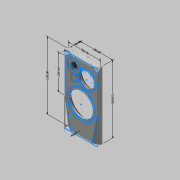
# Autodesk Inventor part: Front-panel
Saved by Autodesk Inventor 2022 (Build 260153070, 153G)
## iProperties
Created: 2021-11-16
Part Number: Front-panel
Material: Типовые
Document SubType Name: Modeling
Designer: kalugin_a
Density: 1 g/cm^3
Appearance: Белый дуб — натуральный — с умеренным глянцем
Author: kalugin_a
Autodesk Inventor part; units mm, degrees
ref_plane "YZ Plane" through (0, 0, 0) normal (1, 0, 0) x (0, 1, 0)
ref_plane "XZ Plane" through (0, 0, 0) normal (0, 1, 0) x (-1, 0, 0)
ref_plane "XY Plane" through (0, 0, 0) normal (0, 0, 1) x (1, 0, 0)
sketch "Эскиз1" plane through (0, 0, 0) normal (0, 0, 1) x (1, 0, 0)
  line L0 (125, 527.1036) -> (125, 6.4626) construction
  circle A0 centre (125, 228.3565) radius 93
  circle A1 centre (168.7833, 413.2707) radius 72.5
  circle A2 centre (67.9786, 456.6783) radius 51
  circle A3 centre (125, 228.3565) radius 110
  line L1 (52.0512, 396.4011) -> (83.9061, 396.4011)
  line L2 (88.9061, 391.4011) -> (88.9061, 359.1741)
  line L3 (83.9061, 354.1741) -> (52.0512, 354.1741)
  line L4 (47.0512, 359.1741) -> (47.0512, 391.4011)
  arc A4 (83.9061, 354.1741) -> (88.9061, 359.1741) centre (83.9061, 359.1741) ccw
  arc A5 (47.0512, 359.1741) -> (52.0512, 354.1741) centre (52.0512, 359.1741) ccw
  arc A6 (52.0512, 396.4011) -> (47.0512, 391.4011) centre (52.0512, 391.4011) ccw
  arc A7 (88.9061, 391.4011) -> (83.9061, 396.4011) centre (83.9061, 391.4011) ccw
  line L5 (0, 7.1036) -> (250, 7.1036)
  line L6 (250, 7.1036) -> (250, 527.1036)
  line L7 (250, 527.1036) -> (0, 527.1036)
  line L8 (0, 527.1036) -> (0, 7.1036)
  circle A8 centre (168.7833, 413.2707) radius 60
  circle A9 centre (67.9786, 456.6783) radius 25
  line L9 (0, 492.1036) -> (45, 527.1036)
  line L10 (205, 527.1036) -> (250, 492.1036)
  line L11 (0, 228.3565) -> (45, 7.1036)
  line L12 (250, 228.3565) -> (205, 7.1036)
  point P0 (106.0245, 471.357)
  point P1 (53.3, 494.7242)
  point P2 (29.9327, 441.9997)
  point P3 (82.6573, 418.6324)
  point P4 (196.0451, 456.6783)
  point P5 (144.8221, 458.584)
  point P6 (117.5603, 415.1763)
  point P7 (141.5215, 369.8631)
  point P8 (192.7445, 367.9575)
  point P9 (220.0063, 411.3651)
  point P10 (125, 328.8295)
  point P11 (53.9549, 299.4016)
  point P12 (24.527, 228.3565)
  point P13 (53.9549, 157.3114)
  point P14 (125, 127.8835)
  point P15 (196.0451, 157.3114)
  point P16 (225.473, 228.3565)
  point P17 (196.0451, 299.4016)
  point P18 (0, 0)
  dimension "d3" = 186
  dimension "d8" = 145
  dimension "d9" = 102
  dimension "d10" = 220
  dimension "d15" = 5
  dimension "d16" = 5
  dimension "d17" = 5
  dimension "d18" = 5
  dimension "d19" = 250
  dimension "d20" = 520
  dimension "d21" = 120
  dimension "d22" = 50
  dimension "d25" = 360
  dimension "d29" = 360
  dimension "d33" = 360
  dimension "d92" = 35
  dimension "d93" = 45
  dimension "d96" = 45
  dimension "d97" = 35
  dimension "d103" = 45
  dimension "d104" = 45
  dimension "d145" = 221.8939
  dimension "d146" = 406.8082
  dimension "d147" = 449.5747
  dimension "d148" = 81.2167
  dimension "d149" = 67.9786
  constraints: 26 end point, 10 centre point, 10 point on line, 8 point on circle, 8 tangent, 3 coincident, 2 parallel, 2 perpendicular, 1 horizontal, 1 midpoint, 1 vertical, 21 other
  measures "d3" diameter of A0
  measures "d8" diameter of A1
  measures "d9" diameter of A2
  measures "d10" diameter of A3
  measures "d15" radius of A4
  measures "d16" radius of A5
  measures "d17" radius of A6
  measures "d18" radius of A7
  measures "d19" distance of L6.end L7.end
  measures "d20" distance of L7.end L5.start
  measures "d21" diameter of A8
  measures "d22" diameter of A9
  measures "d92" distance of L7.end L9.start
  measures "d93" distance from line of L9.end L8
  measures "d96" distance of L10.start L6.end
  measures "d97" distance of L10.end L6.end
  measures "d103" distance of L12.end L5.end
  measures "d104" distance of L11.end L5.start
  measures "d145" distance of A0.centre L0.end
  measures "d146" vertical distance of A8.centre L0.end
  measures "d147" distance from line of L5 A2.centre
  measures "d148" distance from line of L6 A8.centre
  measures "d149" distance from line of L8 A2.centre
extrude "Выдавливание2" add sketch "Эскиз1" against normal blind 40 contours A1 A2 A8 | A2 A8 A1 | A1 A2 | A3 | L1 A7 L2 A4 L3 A5 L4 A6 | L8 L11 L5 | L11 L8 L9 L7 L10 L6 L12 L5 | L12 L6 L5 | L8 L7 L9 | L10 L7 L6
sketch "Эскиз3" plane through (0, 0, 0) normal (0, 0, 1) x (1, 0, 0)
  point P0 (0, 0)
  point P1 (53.2995, 494.7309)
  point P2 (29.4952, 442.4101)
  point P3 (82.4876, 418.8084)
  point P4 (105.644, 471.8009)
  point P5 (127.9097, 465.5665)
  point P6 (193.3079, 474.3405)
  point P7 (233.8339, 422.6329)
  point P8 (209.2871, 361.565)
  point P9 (144.1779, 352.2851)
  point P10 (103.6157, 404.0731)
  point P11 (83.8585, 391.5003)
  point P12 (51.9775, 391.5003)
  point P13 (51.8278, 359.3199)
  point P14 (83.7088, 359.3199)
  point P15 (124.8697, 328.9356)
  point P16 (53.9232, 299.4494)
  point P17 (24.437, 228.3533)
  point P18 (53.9232, 157.4068)
  point P19 (124.8697, 127.7709)
  point P20 (195.9659, 157.4068)
  point P21 (225.4521, 228.503)
  point P22 (195.9659, 299.5991)
hole "Отверстие1" at (53.2995, 494.7309, 0) at (29.4952, 442.4101, 0) at (82.4876, 418.8084, 0) at (105.644, 471.8009, 0) at (127.9097, 465.5665, 0) at (193.3079, 474.3405, 0) at (233.8339, 422.6329, 0) at (209.2871, 361.565, 0) at (144.1779, 352.2851, 0) at (103.6157, 404.0731, 0) at (83.8585, 391.5003, 0) at (51.9775, 391.5003, 0) at (51.8278, 359.3199, 0) at (83.7088, 359.3199, 0) at (124.8697, 328.9356, 0) at (53.9232, 299.4494, 0) at (24.437, 228.3533, 0) at (53.9232, 157.4068, 0) at (124.8697, 127.7709, 0) at (195.9659, 157.4068, 0) at (225.4521, 228.503, 0) at (195.9659, 299.5991, 0) direction (0, 0, -1) diameter 5 end through all counterbore diameter 6 counterbore depth 5
sketch "Эскиз4" plane through (0, 0, 0) normal (0, 0, 1) x (1, 0, 0)
  circle A0 centre (124.9966, 228.3645) radius 109.8136
  circle A1 centre (168.7833, 413.2703) radius 72.3983
  circle A2 centre (67.9786, 456.6783) radius 50.8827
  point P0 (0, 0)
  point P1 (118.17, 465.0372)
  point P2 (96.395, 414.4698)
  constraints: 3 centre point
extrude "Выдавливание3" cut sketch "Эскиз4" against normal blind 4
sketch "Эскиз6" plane through (0, 0, -4) normal (0, 0, 1) x (1, 0, 0)
  point P0 (0, 0)
  point P1 (78.9885, 479.1235)
  dimension "d3" = 186
  dimension "d8" = 145
  dimension "d9" = 102
  dimension "d10" = 220
  dimension "d19" = 250
  dimension "d20" = 520
  dimension "d21" = 120
  dimension "d22" = 50
  dimension "d25" = 360
  dimension "d29" = 360
  dimension "d33" = 360
  dimension "d92" = 35
  dimension "d93" = 45
  dimension "d96" = 45
  dimension "d97" = 35
  dimension "d103" = 45
  dimension "d104" = 45
  dimension "d145" = 221.8939
  dimension "d146" = 406.8082
  dimension "d147" = 449.5747
  dimension "d148" = 81.2167
  dimension "d149" = 67.9786
hole "Отверстие3" at (78.9885, 479.1235, -4) direction (0, 0, -1) diameter 15 end through all
sketch "Эскиз7" plane through (0, 0, -4) normal (0, 0, 1) x (1, 0, 0)
  point P0 (0, 0)
  point P1 (58.1005, 433.7127)
hole "Отверстие4" at (58.1005, 433.7127, -4) direction (0, 0, -1) diameter 15 end through all
sketch "Эскиз8" plane through (0, 0, 0) normal (0, 0, 1) x (1, 0, 0)
  line L0 (52.0512, 396.4011) -> (83.9061, 396.4011)
  line L1 (88.9061, 391.4011) -> (88.9061, 359.1741)
  line L2 (83.9061, 354.1741) -> (52.0512, 354.1741)
  line L3 (47.0512, 359.1741) -> (47.0512, 391.4011)
  arc A0 (83.9061, 354.1741) -> (88.9061, 359.1741) centre (83.9061, 359.1741) ccw
  arc A1 (47.0512, 359.1741) -> (52.0512, 354.1741) centre (52.0512, 359.1741) ccw
  arc A2 (52.0512, 396.4011) -> (47.0512, 391.4011) centre (52.0512, 391.4011) ccw
  arc A3 (88.9061, 391.4011) -> (83.9061, 396.4011) centre (83.9061, 391.4011) ccw
  point P0 (0, 0)
  point P1 (125, 228.3565)
  point P2 (168.7833, 413.2707)
  point P3 (67.9786, 456.6783)
  point P4 (106.0245, 471.357)
  point P5 (53.3, 494.7242)
  point P6 (29.9327, 441.9997)
  point P7 (82.6573, 418.6324)
  point P8 (128.1827, 465.0454)
  point P9 (103.6449, 403.9969)
  point P10 (144.2455, 352.2222)
  point P11 (209.3839, 361.4961)
  point P12 (233.9218, 422.5446)
  point P13 (193.3212, 474.3192)
  point P14 (125, 328.8295)
  point P15 (53.9549, 299.4016)
  point P16 (24.527, 228.3565)
  point P17 (53.9549, 157.3114)
  point P18 (125, 127.8835)
  point P19 (196.0451, 157.3114)
  point P20 (225.473, 228.3565)
  point P21 (196.0451, 299.4016)
  point P22 (0, 0)
  dimension "d77" = 5
  dimension "d78" = 5
  dimension "d79" = 5
  dimension "d80" = 5
  dimension "d85" = 360
  dimension "d86" = 360
  dimension "d87" = 360
  constraints: 8 end point, 8 point on circle, 8 tangent, 4 centre point, 1 perpendicular, 21 other
  measures "d77" radius of A0
  measures "d78" radius of A1
  measures "d79" radius of A2
  measures "d80" radius of A3
extrude "Выдавливание4" cut sketch "Эскиз8" against normal blind 2
sketch "Эскиз9" plane through (0, 7.1036, 0) normal (-1, 0, 0) x (0, 0, 1)
  line L0 (0, 520) -> (-40, 520) projected
  line L1 (-25, 520) -> (0, 485)
  point P0 (0, -7.1036)
  dimension "d90" = 35
  dimension "d91" = 25
  constraints: 2 end point, 1 point on line
  measures "d90" distance of L0.start L1.end
  measures "d91" distance of L0.start L1.start
sketch "Эскиз10" plane through (0, 527.1036, 0) normal (0, 1, 0) x (1, 0, 0)
  line L0 (0, 0) -> (0, 40) projected
  line L1 (0, 25) -> (45, 0)
  line L2 (250, 0) -> (0, 0) projected
  dimension "d94" = 45
  dimension "d95" = 25
  constraints: 2 end point, 2 point on line
  measures "d94" distance from line of L1.end L0
  measures "d95" distance of L1.start L0.start
ref_plane "РабПлоскость1" through (45, 527.1036, 0) normal (0.4119358, -0.5296317, -0.7414844) x (-0.7893522, -0.6139406, 0)
split "Разделение1" plane through (45, 527.1036, 0) removes the side toward (-0.4119358, 0.5296317, 0.7414844)
sketch "Эскиз11" plane through (250, 7.1036, 0) normal (1, 0, 0) x (0, 0, -1)
  line L0 (0, 520) -> (40, 520) projected
  line L1 (0, 398.6921) -> (0, 500.4574) projected
  point P0 (0, -7.1036)
  point P1 (25, 520)
  point P2 (0, 485)
  point P3 (0, 407.3662)
  point P4 (0, 457.9336)
  dimension "d98" = 25
  dimension "d99" = 35
  constraints: 2 point on line
  measures "d98" distance of point (25, 520) L0.start
  measures "d99" distance of point (0, 485) L0.start
sketch "Эскиз12" plane through (0, 527.1036, -40) normal (0, 1, 0) x (1, 0, 0)
  line L0 (0, -40) -> (250, -40) projected
  point P0 (205, -40)
  dimension "d100" = 45
  constraints: 1 point on line
  measures "d100" distance of point (205, -40) L0.end
ref_plane "РабПлоскость2" through (250, 527.1036, -25) normal (-0.4119358, -0.5296317, -0.7414844) x (0, -0.8137335, 0.5812382)
split "Разделение2" plane through (250, 527.1036, -25) removes the side toward (0.4119358, 0.5296317, 0.7414844)
sketch "Эскиз13" plane through (250, 7.1036, -40) normal (1, 0, 0) x (0, 0, -1)
  line L0 (-39.9472, 218.8994) -> (-15, 0)
  line L1 (-40, 0) -> (0, 0) projected
  point P0 (-40, -7.1036)
  dimension "d101" = 25
  constraints: 2 end point, 1 point on line
  measures "d101" distance of L0.end L1.start
sketch "Эскиз14" plane through (0, 0, 0) normal (0, 0, 1) x (1, 0, 0)
  point P0 (0, 0)
sketch "Эскиз15" plane through (0, 7.1036, 0) normal (0, -1, 0) x (1, 0, 0)
  line L0 (250, -25) -> (250, -40) projected
  line L1 (205, 0) -> (250, -25) projected
  line L2 (250, -25) -> (205, 0)
  line L3 (0, -25) -> (45, 0) projected
  line L4 (45, 0) -> (0, -25)
  point P0 (0, 0)
  dimension "d102" = 25
  constraints: 4 end point, 2 collinear
  measures "d102" distance of L3.start point (0, 0)
ref_plane "РабПлоскость3" through (250, 226.003, -0.0528) normal (-0.4832507, 0.0991339, -0.8698513) x (0, -0.9935684, -0.1132336)
split "Разделение3" plane through (250, 226.003, -0.0528) removes the side toward (0.4832507, -0.0991339, 0.8698513)
sketch "Эскиз16" plane through (0, 7.1036, -40) normal (-1, 0, 0) x (0, 0, 1)
  line L0 (40, 219.3626) -> (15, 0) projected
  point P0 (40, -7.1036)
ref_plane "РабПлоскость4" through (0, 226.4662, 0) normal (0.4832507, 0.0991339, -0.8698513) x (0.200955, -0.9796005, 0)
split "Разделение4" plane through (0, 226.4662, 0) removes the side toward (-0.4832507, -0.0991339, 0.8698513)
chamfer "Фаска1" distance 7 angle 45 1 edges at (125, 527.1036, 0)
chamfer "Фаска2" distance 7 angle 45 1 edges at (125, 7.1036, 0)
chamfer "Фаска3" distance 25 angle 45 1 edges at (32, 228.3565, -40)
chamfer "Фаска4" distance 20 angle 45 1 edges at (108.7833, 413.2707, -40)
